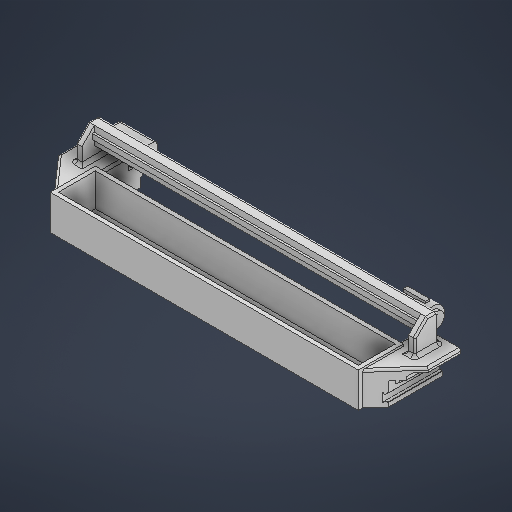
# Autodesk Inventor part: SACMI PH1500 HOPPER FEEDER
Saved by Autodesk Inventor 2025 (Build 290162000, 162)
## iProperties
Created: 2024-05-04
Part Number: SACMI PH1500 HOPPER FEEDER
Material: Generic
Document SubType Name: Modeling
Designer: zulet
Density: 1 g/cm^3
Appearance: Default
Author: zulet
Autodesk Inventor part; units mm, degrees
ref_plane "YZ Plane" through (0, 0, 0) normal (1, 0, 0) x (0, 1, 0)
ref_plane "XZ Plane" through (0, 0, 0) normal (0, 1, 0) x (-1, 0, 0)
ref_plane "XY Plane" through (0, 0, 0) normal (0, 0, 1) x (1, 0, 0)
sketch "Sketch1" plane through (0, 0, 0) normal (0, 1, 0) x (-1, 0, 0)
  line L0 (750, -110) -> (-750, -110)
  line L1 (-750, -110) -> (-750, 110)
  line L2 (-750, 110) -> (750, 110)
  line L3 (750, 110) -> (750, -110)
  line L4 (750, -110) -> (-750, 110) construction
  line L5 (-750, -110) -> (750, 110) construction
  line L6 (-730, -90) -> (730, -90)
  line L7 (730, -90) -> (730, 90)
  line L8 (730, 90) -> (-730, 90)
  line L9 (-730, 90) -> (-730, -90)
  line L10 (-750, 90) -> (-900, -80)
  line L11 (-900, -80) -> (-900, -240)
  line L12 (-900, -240) -> (-720, -240)
  line L13 (-720, -240) -> (-720, -110)
  point P0 (0, 0)
  dimension "d0" = 1500
  dimension "d1" = 220
  dimension "d2" = 20
  dimension "d7" = 150
  dimension "d8" = 20
  dimension "d9" = 30
  dimension "d10" = 130
  dimension "d11" = 30
  constraints: 28 end point, 4 parallel, 4 perpendicular, 2 midpoint, 2 point on line, 1 horizontal, 1 vertical, 3 other
  measures "d0" distance of L1.end L2.end
  measures "d1" distance of L0.end L1.end
  measures "d2" distance between parallel lines of L0 L6
  measures "d7" distance between parallel lines of L11 L1
  measures "d8" distance from line of L2 L10.start
  measures "d9" distance from line of L10.end L0
  measures "d10" distance between parallel lines of L0 L12
  measures "d11" distance between parallel lines of L1 L13
extrude "Extrusion1" add sketch "Sketch1" along normal blind 10 contours L9 L8 L7 L6
extrude "Extrusion2" add sketch "Sketch1" along normal blind 170 contours L0 L1 L2 L3
extrude "Extrusion3" add sketch "Sketch1" along normal blind 160 contours L13 L12 L11 L10 L1 L0
sketch "Sketch2" plane through (900, 0, -240) normal (0, 0, -1) x (-1, 0, 0)
  line L0 (150, 0) -> (0, 0) projected
  line L1 (90, 110) -> (50, 110)
  line L2 (50, 125) -> (35, 140)
  line L3 (35, 140) -> (0, 140)
  line L4 (0, 160) -> (180, 160) projected
  line L5 (0, 0) -> (180, 0) projected
  line L6 (180, 0) -> (180, 160) projected
  line L7 (0, 160) -> (180, 160) projected
  line L8 (0, 0) -> (0, 160) projected
  line L9 (90, 110) -> (90, 0)
  line L10 (65, 110) -> (75, 110)
  line L11 (75, 110) -> (75, 100)
  line L12 (75, 100) -> (65, 100)
  line L13 (65, 100) -> (65, 110)
  line L14 (90, 20) -> (105, 20)
  line L15 (105, 20) -> (105, 60)
  line L16 (105, 60) -> (90, 60)
  line L17 (90, 60) -> (90, 20)
  circle A0 centre (97.5, 60) radius 5
  circle A1 centre (97.5, 20) radius 5
  line L18 (50, 125) -> (50, 110)
  point P0 (900, 0)
  point P1 (70, 110)
  point P2 (90, 20)
  point P3 (92.5, 20)
  point P4 (102.5, 20)
  point P5 (102.5, 60)
  point P6 (92.5, 60)
  point P7 (90, 75.9726)
  point P8 (75, 110)
  point P9 (65, 110)
  point P10 (75, 110)
  dimension "d14" = 20
  dimension "d15" = 35
  dimension "d16" = 15
  dimension "d17" = 15
  dimension "d18" = 40
  dimension "d19" = 10
  dimension "d20" = 10
  dimension "d21" = 15
  dimension "d22" = 40
  dimension "d23" = 10
  dimension "d24" = 10
  dimension "d28" = 15
  dimension "d29" = 50
  constraints: 26 end point, 5 midpoint, 5 parallel, 2 centre point, 2 horizontal, 2 perpendicular, 2 point on line, 1 vertical
  measures "d14" distance between parallel lines of L4 L3
  measures "d15" distance of L2.end L3.end
  measures "d16" horizontal distance of L2.start L2.end
  measures "d17" horizontal distance of L2.start L2.end
  measures "d18" distance of L1.start L1.end
  measures "d19" distance of L11.end L12.end
  measures "d20" distance of L10.end L11.end
  measures "d21" distance of L15.end L16.end
  measures "d22" distance of L14.end L15.end
  measures "d23" diameter of A0
  measures "d24" diameter of A1
  measures "d28" distance of L2.start L1.end
  measures "d29" distance between parallel lines of L1 L16
extrude "Extrusion4" cut sketch "Sketch2" against normal through all contours L0 L8 L3 L2 L18 L1 L13 L12 L11 L9 | L9 L16 A0 L15 L14 A1
fillet "Fillet1" radius 10 3 edges at (825, 160, 5) (900, 160, -160) (720, 160, -175)
mirror "Mirror1" about plane through (0, 0, 0) normal (1, 0, 0) of "Extrusion3", "Extrusion4", "Fillet1"
sketch "Sketch3" plane through (0, 160, 0) normal (0, 1, 0) x (1, 0, 0)
  line L0 (795, 205) -> (825, 205)
  line L1 (825, 205) -> (825, 90)
  line L2 (825, 90) -> (795, 90)
  line L3 (795, 90) -> (795, 205)
  line L4 (890, 240) -> (730, 240) construction
  line L5 (810, 240) -> (810, -10) construction
  line L6 (807.5, 240) -> (807.5, -24.8333) construction
  line L7 (810, 240) -> (1060, 240) construction
  point P0 (0, 0)
  point P1 (810, 205)
  dimension "d30" = 30
  dimension "d31" = 115
  dimension "d32" = 250
  dimension "d33" = 90
  dimension "d34" = 35
  constraints: 12 end point, 3 parallel, 2 horizontal, 2 midpoint, 2 perpendicular, 1 point on line
  measures "d30" distance of L1.end L2.end
  measures "d31" distance of L0.end L1.end
  measures "d32" distance of L5.start L5.end
  measures "d33" angle of L5 L7
  measures "d34" distance between parallel lines of L4 L0
extrude "Extrusion5" add sketch "Sketch3" along normal blind 140
chamfer "Chamfer1" distance 60 angle 45 1 edges at (810, 300, -90)
fillet "Fillet2" radius 8 4 edges at (825, 300, -177.5) (825, 270, -120) (825, 200, -90) (825, 230, -205)
fillet "Fillet3" radius 15 6 edges at (822.6569, 160, -92.3431) (806, 160, -90) (822.6569, 160, -202.6569) (806, 160, -205) (825, 160, -147.5) (795, 160, -147.5)
mirror "Mirror2" about plane through (0, 0, 0) normal (1, 0, 0) of "Extrusion5", "Chamfer1", "Fillet2", "Fillet3"
sketch "Sketch4" plane through (-795, 175, -205) normal (1, 0, 0) x (0, 0, -1)
  line L0 (0, 0) -> (-115, 0) projected
  line L1 (0, 0) -> (0, 125) projected
  line L2 (0, 125) -> (-55, 125) projected
  line L3 (-55, 125) -> (-115, 65) projected
  line L4 (-115, 0) -> (-115, 65) projected
  line L5 (0, 125) -> (0, 0) projected
  line L6 (-55, 125) -> (0, 125)
  line L7 (0, 125) -> (0, 40)
  line L8 (0, 40) -> (-55, 40)
  line L9 (-55, 40) -> (-55, 125)
  line L10 (-55, 95) -> (-65, 95)
  line L11 (-65, 95) -> (-65, 70)
  line L12 (-65, 70) -> (-55, 70)
  line L13 (-55, 70) -> (-55, 95)
  point P0 (-205, -175)
  point P1 (-55, 82.5)
  point P2 (-55, 70)
  point P3 (-55, 95)
  dimension "d42" = 85
  dimension "d45" = 10
  dimension "d46" = 25
  constraints: 16 end point, 4 parallel, 2 horizontal, 2 midpoint, 2 perpendicular, 1 point on line
  measures "d42" distance of L8.end L2.end
  measures "d45" distance of L12.end L11.end
  measures "d46" distance of L11.end L10.end
extrude "Extrusion6" add sketch "Sketch4" along normal up to surface (1590 mm away) contours L8 L9 L2 L1 | L12 L11 L10 L9
chamfer "Chamfer2" distance 30 angle 45 1 edges at (0, 215, -205)
fillet "Fillet4" radius 15 3 edges at (-822.6569, 297.6569, -202.6569) (822.6569, 297.6569, -202.6569) (0, 300, -205)
sketch "Sketch5" plane through (-720, 0, -240) normal (0, 0, -1) x (-1, 0, 0)
  line L0 (-1440, 150) -> (-1440, 0) projected
  line L1 (-1440, 0) -> (-1470, 0)
  line L2 (-1470, 0) -> (-1470, 100)
  line L3 (-1470, 100) -> (-1440, 100)
  line L4 (-1440, 100) -> (-1440, 0)
  line L5 (90, 0) -> (0, 0) projected
  line L6 (0, 0) -> (30, 0)
  line L7 (30, 0) -> (30, 100)
  line L8 (30, 100) -> (0, 100)
  line L9 (0, 100) -> (0, 0)
  point P0 (-720, 0)
  dimension "d51" = 30
  dimension "d52" = 100
  dimension "d53" = 30
  dimension "d54" = 100
  constraints: 16 end point, 4 parallel, 2 horizontal, 2 perpendicular
  measures "d51" distance of L2.end L3.end
  measures "d52" distance of L1.end L2.end
  measures "d53" distance of L8.end L7.end
  measures "d54" distance of L7.end L6.end
extrude "Extrusion7" add sketch "Sketch5" along normal blind 60
sketch "Sketch6" plane through (-720, 0, -300) normal (0, 0, -1) x (-1, 0, 0)
  line L0 (180, 160) -> (0, 160)
  line L1 (0, 160) -> (0, 80)
  line L2 (0, 80) -> (180, 80)
  line L3 (180, 80) -> (180, 160)
  line L4 (170, 160) -> (10, 160) projected
  line L5 (180, 140) -> (180, 150) projected
  point P0 (-720, 0)
  dimension "d57" = 180
  dimension "d58" = 80
  constraints: 8 end point, 2 collinear, 2 parallel, 1 horizontal, 1 perpendicular
  measures "d57" distance of L2.end L1.end
  measures "d58" distance of L1.end L0.end
extrude "Extrusion8" add sketch "Sketch6" along normal blind 80
fillet "Fillet5" radius 15 8 edges at (-810, 160, -380) (-900, 160, -340) (-810, 160, -300) (-900, 120, -300) (-900, 120, -380) (-900, 80, -340) (-810, 80, -380) (-825, 80, -300)
chamfer "Chamfer3" distance 40 angle 45 1 edges at (-735, 100, -300)
chamfer "Chamfer4" distance 40 angle 45 1 edges at (-735, 80, -300)
fillet "Fillet6" radius 10 3 edges at (-750, 84.3934, -304.3934) (-750, 80, -327.5) (-750, 117.5, -300)
sketch "Sketch7" plane through (-720, 0, -110) normal (1, 0, 0) x (0, 0, -1)
  line L0 (205, 145) -> (205, 95) projected
  line L1 (255, 95) -> (255, 80) projected
  line L2 (205, 145) -> (255, 95) construction
  line L3 (255, 145) -> (270, 145) projected
  line L4 (205, 95) -> (255, 95) projected
  line L5 (255, 145) -> (205, 95) construction
  circle A0 centre (230, 120) radius 25
  line L6 (255, 145) -> (205, 145) projected
  point P0 (-110, 0)
  constraints: 4 end point, 1 centre point, 1 midpoint, 1 tangent
extrude "Extrusion9" add sketch "Sketch7" along normal blind 1250 contours A0
sketch "Sketch8" plane through (530, 120, -340) normal (1, 0, 0) x (0, 0, -1)
  circle A0 centre (0, 0) radius 25 projected
  circle A1 centre (0, 0) radius 50
  point P0 (-340, -120)
  dimension "d71" = 100
  constraints: 1 centre point, 1 coincident
  measures "d71" diameter of A1
extrude "Extrusion10" add sketch "Sketch8" along normal blind 15 contours A0 | A1
sketch "Sketch9" plane through (545, 120, -340) normal (1, 0, 0) x (0, 0, -1)
  circle A0 centre (0, 0) radius 50 projected
  line L0 (2, 57.5) -> (-2, 57.5)
  line L1 (-2, 57.5) -> (-2, 44.5)
  line L2 (0, 42.5) -> (0, 42.5)
  line L3 (2, 44.5) -> (2, 57.5)
  line L4 (2, 57.5) -> (-2, 42.5) construction
  line L5 (-2, 57.5) -> (2, 42.5) construction
  arc A1 (-2, 44.5) -> (0, 42.5) centre (0, 44.5) ccw
  arc A2 (0, 42.5) -> (2, 44.5) centre (0, 44.5) ccw
  line L6 (-12.2349, 56.2188) -> (-9.9136, 43.4278)
  arc A3 (-9.9136, 43.4278) -> (-7.5887, 41.817) centre (-7.9458, 43.7849) ccw
  arc A4 (-7.5887, 41.817) -> (-5.9779, 44.142) centre (-7.9458, 43.7849) ccw
  line L7 (-5.9779, 44.142) -> (-8.2992, 56.9331)
  line L8 (-8.2992, 56.9331) -> (-12.2349, 56.2188)
  line L9 (-22.0765, 53.1308) -> (-17.5086, 40.9597)
  arc A5 (-17.5086, 40.9597) -> (-14.9334, 39.79) centre (-15.6362, 41.6625) ccw
  arc A6 (-14.9334, 39.79) -> (-13.7637, 42.3652) centre (-15.6362, 41.6625) ccw
  line L10 (-13.7637, 42.3652) -> (-18.3316, 54.5363)
  line L11 (-18.3316, 54.5363) -> (-22.0765, 53.1308)
  line L12 (-31.2086, 48.335) -> (-24.5409, 37.1752)
  arc A7 (-24.5409, 37.1752) -> (-21.7982, 36.4841) centre (-22.824, 38.201) ccw
  arc A8 (-21.7982, 36.4841) -> (-21.1071, 39.2268) centre (-22.824, 38.201) ccw
  line L13 (-21.1071, 39.2268) -> (-27.7748, 50.3866)
  line L14 (-27.7748, 50.3866) -> (-31.2086, 48.335)
  line L15 (-39.3376, 41.9857) -> (-30.7844, 32.1958)
  arc A9 (-30.7844, 32.1958) -> (-27.9624, 32.0055) centre (-29.2783, 33.5117) ccw
  arc A10 (-27.9624, 32.0055) -> (-27.7721, 34.8276) centre (-29.2783, 33.5117) ccw
  line L16 (-27.7721, 34.8276) -> (-36.3253, 44.6175)
  line L17 (-36.3253, 44.6175) -> (-39.3376, 41.9857)
  line L18 (-46.2023, 34.287) -> (-36.0385, 26.1816)
  arc A11 (-36.0385, 26.1816) -> (-33.2278, 26.4983) centre (-34.7915, 27.7453) ccw
  arc A12 (-33.2278, 26.4983) -> (-33.5445, 29.309) centre (-34.7915, 27.7453) ccw
  line L19 (-33.5445, 29.309) -> (-43.7083, 37.4143)
  line L20 (-43.7083, 37.4143) -> (-46.2023, 34.287)
  line L21 (-51.582, 25.4863) -> (-40.1342, 19.326)
  arc A13 (-40.1342, 19.326) -> (-37.4253, 20.1394) centre (-39.1865, 21.0872) ccw
  arc A14 (-37.4253, 20.1394) -> (-38.2388, 22.8483) centre (-39.1865, 21.0872) ccw
  line L22 (-38.2388, 22.8483) -> (-49.6865, 29.0086)
  line L23 (-49.6865, 29.0086) -> (-51.582, 25.4863)
  line L24 (-55.3038, 15.8664) -> (-42.94, 11.8491)
  arc A15 (-42.94, 11.8491) -> (-40.4199, 13.1332) centre (-42.322, 13.7513) ccw
  arc A16 (-40.4199, 13.1332) -> (-41.704, 15.6534) centre (-42.322, 13.7513) ccw
  line L25 (-41.704, 15.6534) -> (-54.0677, 19.6706)
  line L26 (-54.0677, 19.6706) -> (-55.3038, 15.8664)
  line L27 (-57.2481, 5.7365) -> (-44.3657, 3.9915)
  arc A17 (-44.3657, 3.9915) -> (-42.1154, 5.7049) centre (-44.0973, 5.9734) ccw
  arc A18 (-42.1154, 5.7049) -> (-43.8288, 7.9553) centre (-44.0973, 5.9734) ccw
  line L28 (-43.8288, 7.9553) -> (-56.7111, 9.7003)
  line L29 (-56.7111, 9.7003) -> (-57.2481, 5.7365)
  line L30 (-57.3524, -4.5777) -> (-44.3655, -3.9945)
  arc A19 (-44.3655, -3.9945) -> (-42.4572, -1.9068) centre (-44.4552, -1.9965) ccw
  arc A20 (-42.4572, -1.9068) -> (-44.5449, 0.0015) centre (-44.4552, -1.9965) ccw
  line L31 (-44.5449, 0.0015) -> (-57.5318, -0.5817)
  line L32 (-57.5318, -0.5817) -> (-57.3524, -4.5777)
  line L33 (-55.6133, -14.7448) -> (-42.9393, -11.852)
  arc A21 (-42.9393, -11.852) -> (-41.4344, -9.4571) centre (-43.3843, -9.9022) ccw
  arc A22 (-41.4344, -9.4571) -> (-43.8293, -7.9523) centre (-43.3843, -9.9022) ccw
  line L34 (-43.8293, -7.9523) -> (-56.5034, -10.8451)
  line L35 (-56.5034, -10.8451) -> (-55.6133, -14.7448)
  line L36 (-52.0868, -24.438) -> (-40.1329, -19.3287)
  arc A23 (-40.1329, -19.3287) -> (-39.0799, -16.7036) centre (-40.919, -17.4896) ccw
  arc A24 (-39.0799, -16.7036) -> (-41.705, -15.6506) centre (-40.919, -17.4896) ccw
  line L37 (-41.705, -15.6506) -> (-53.6589, -20.7599)
  line L38 (-53.6589, -20.7599) -> (-52.0868, -24.438)
  line L39 (-46.8862, -33.3457) -> (-36.0367, -26.1841)
  arc A25 (-36.0367, -26.1841) -> (-35.4694, -23.4131) centre (-37.1385, -24.5149) ccw
  arc A26 (-35.4694, -23.4131) -> (-38.2403, -22.8458) centre (-37.1385, -24.5149) ccw
  line L40 (-38.2403, -22.8458) -> (-49.0898, -30.0074)
  line L41 (-49.0898, -30.0074) -> (-46.8862, -33.3457)
  line L42 (-40.1786, -41.1817) -> (-30.7822, -32.1979)
  arc A27 (-30.7822, -32.1979) -> (-30.7188, -29.3702) centre (-32.1644, -30.7523) ccw
  arc A28 (-30.7188, -29.3702) -> (-33.5465, -29.3067) centre (-32.1644, -30.7523) ccw
  line L43 (-33.5465, -29.3067) -> (-42.9428, -38.2905)
  line L44 (-42.9428, -38.2905) -> (-40.1786, -41.1817)
  line L45 (-32.1796, -47.694) -> (-24.5384, -37.1768)
  arc A29 (-24.5384, -37.1768) -> (-24.9809, -34.3832) centre (-26.1564, -36.0013) ccw
  arc A30 (-24.9809, -34.3832) -> (-27.7745, -34.8257) centre (-26.1564, -36.0013) ccw
  line L46 (-27.7745, -34.8257) -> (-35.4157, -45.3429)
  line L47 (-35.4157, -45.3429) -> (-32.1796, -47.694)
  line L48 (-23.1464, -52.6735) -> (-17.5059, -40.9609)
  arc A31 (-17.5059, -40.9609) -> (-18.4401, -38.2912) centre (-19.3078, -40.0931) ccw
  arc A32 (-18.4401, -38.2912) -> (-21.1098, -39.2253) centre (-19.3078, -40.0931) ccw
  line L49 (-21.1098, -39.2253) -> (-26.7503, -50.9379)
  line L50 (-26.7503, -50.9379) -> (-23.1464, -52.6735)
  line L51 (-13.3692, -55.9599) -> (-9.9107, -43.4284)
  arc A33 (-9.9107, -43.4284) -> (-11.3066, -40.9684) centre (-11.8386, -42.8963) ccw
  arc A34 (-11.3066, -40.9684) -> (-13.7666, -42.3643) centre (-11.8386, -42.8963) ccw
  line L52 (-13.7666, -42.3643) -> (-17.225, -54.8958)
  line L53 (-17.225, -54.8958) -> (-13.3692, -55.9599)
  line L54 (-3.1623, -57.4478) -> (-1.997, -44.5001)
  arc A35 (-1.997, -44.5001) -> (-3.8097, -42.3289) centre (-3.9889, -44.3209) ccw
  arc A36 (-3.8097, -42.3289) -> (-5.9809, -44.1416) centre (-3.9889, -44.3209) ccw
  line L55 (-5.9809, -44.1416) -> (-7.1462, -57.0892)
  line L56 (-7.1462, -57.0892) -> (-3.1623, -57.4478)
  line L57 (7.1462, -57.0892) -> (5.9809, -44.1416)
  arc A37 (5.9809, -44.1416) -> (3.8097, -42.3289) centre (3.9889, -44.3209) ccw
  arc A38 (3.8097, -42.3289) -> (1.997, -44.5001) centre (3.9889, -44.3209) ccw
  line L58 (1.997, -44.5001) -> (3.1623, -57.4478)
  line L59 (3.1623, -57.4478) -> (7.1462, -57.0892)
  line L60 (17.225, -54.8958) -> (13.7666, -42.3643)
  arc A39 (13.7666, -42.3643) -> (11.3066, -40.9684) centre (11.8386, -42.8963) ccw
  arc A40 (11.3066, -40.9684) -> (9.9107, -43.4284) centre (11.8386, -42.8963) ccw
  line L61 (9.9107, -43.4284) -> (13.3692, -55.9599)
  line L62 (13.3692, -55.9599) -> (17.225, -54.8958)
  line L63 (26.7503, -50.9379) -> (21.1098, -39.2253)
  arc A41 (21.1098, -39.2253) -> (18.4401, -38.2912) centre (19.3078, -40.0931) ccw
  arc A42 (18.4401, -38.2912) -> (17.5059, -40.9609) centre (19.3078, -40.0931) ccw
  line L64 (17.5059, -40.9609) -> (23.1464, -52.6735)
  line L65 (23.1464, -52.6735) -> (26.7503, -50.9379)
  line L66 (35.4157, -45.3429) -> (27.7745, -34.8257)
  arc A43 (27.7745, -34.8257) -> (24.9809, -34.3832) centre (26.1564, -36.0013) ccw
  arc A44 (24.9809, -34.3832) -> (24.5384, -37.1768) centre (26.1564, -36.0013) ccw
  line L67 (24.5384, -37.1768) -> (32.1796, -47.694)
  line L68 (32.1796, -47.694) -> (35.4157, -45.3429)
  line L69 (42.9428, -38.2905) -> (33.5465, -29.3067)
  arc A45 (33.5465, -29.3067) -> (30.7188, -29.3702) centre (32.1644, -30.7523) ccw
  arc A46 (30.7188, -29.3702) -> (30.7822, -32.1979) centre (32.1644, -30.7523) ccw
  line L70 (30.7822, -32.1979) -> (40.1786, -41.1817)
  line L71 (40.1786, -41.1817) -> (42.9428, -38.2905)
  line L72 (49.0898, -30.0074) -> (38.2403, -22.8458)
  arc A47 (38.2403, -22.8458) -> (35.4694, -23.4131) centre (37.1385, -24.5149) ccw
  arc A48 (35.4694, -23.4131) -> (36.0367, -26.1841) centre (37.1385, -24.5149) ccw
  line L73 (36.0367, -26.1841) -> (46.8862, -33.3457)
  line L74 (46.8862, -33.3457) -> (49.0898, -30.0074)
  line L75 (53.6589, -20.7599) -> (41.705, -15.6506)
  arc A49 (41.705, -15.6506) -> (39.0799, -16.7036) centre (40.919, -17.4896) ccw
  arc A50 (39.0799, -16.7036) -> (40.1329, -19.3287) centre (40.919, -17.4896) ccw
  line L76 (40.1329, -19.3287) -> (52.0868, -24.438)
  line L77 (52.0868, -24.438) -> (53.6589, -20.7599)
  line L78 (56.5034, -10.8451) -> (43.8293, -7.9523)
  arc A51 (43.8293, -7.9523) -> (41.4344, -9.4571) centre (43.3843, -9.9022) ccw
  arc A52 (41.4344, -9.4571) -> (42.9393, -11.852) centre (43.3843, -9.9022) ccw
  line L79 (42.9393, -11.852) -> (55.6133, -14.7448)
  line L80 (55.6133, -14.7448) -> (56.5034, -10.8451)
  line L81 (57.5318, -0.5817) -> (44.5449, 0.0015)
  arc A53 (44.5449, 0.0015) -> (42.4572, -1.9068) centre (44.4552, -1.9965) ccw
  arc A54 (42.4572, -1.9068) -> (44.3655, -3.9945) centre (44.4552, -1.9965) ccw
  line L82 (44.3655, -3.9945) -> (57.3524, -4.5777)
  line L83 (57.3524, -4.5777) -> (57.5318, -0.5817)
  line L84 (56.7111, 9.7003) -> (43.8288, 7.9553)
  arc A55 (43.8288, 7.9553) -> (42.1154, 5.7049) centre (44.0973, 5.9734) ccw
  arc A56 (42.1154, 5.7049) -> (44.3657, 3.9915) centre (44.0973, 5.9734) ccw
  line L85 (44.3657, 3.9915) -> (57.2481, 5.7365)
  line L86 (57.2481, 5.7365) -> (56.7111, 9.7003)
  line L87 (54.0677, 19.6706) -> (41.704, 15.6534)
  arc A57 (41.704, 15.6534) -> (40.4199, 13.1332) centre (42.322, 13.7513) ccw
  arc A58 (40.4199, 13.1332) -> (42.94, 11.8491) centre (42.322, 13.7513) ccw
  line L88 (42.94, 11.8491) -> (55.3038, 15.8664)
  line L89 (55.3038, 15.8664) -> (54.0677, 19.6706)
  line L90 (49.6865, 29.0086) -> (38.2388, 22.8483)
  arc A59 (38.2388, 22.8483) -> (37.4253, 20.1394) centre (39.1865, 21.0872) ccw
  arc A60 (37.4253, 20.1394) -> (40.1342, 19.326) centre (39.1865, 21.0872) ccw
  line L91 (40.1342, 19.326) -> (51.582, 25.4863)
  line L92 (51.582, 25.4863) -> (49.6865, 29.0086)
  line L93 (43.7083, 37.4143) -> (33.5445, 29.309)
  arc A61 (33.5445, 29.309) -> (33.2278, 26.4983) centre (34.7915, 27.7453) ccw
  arc A62 (33.2278, 26.4983) -> (36.0385, 26.1816) centre (34.7915, 27.7453) ccw
  line L94 (36.0385, 26.1816) -> (46.2023, 34.287)
  line L95 (46.2023, 34.287) -> (43.7083, 37.4143)
  line L96 (36.3253, 44.6175) -> (27.7721, 34.8276)
  arc A63 (27.7721, 34.8276) -> (27.9624, 32.0055) centre (29.2783, 33.5117) ccw
  arc A64 (27.9624, 32.0055) -> (30.7844, 32.1958) centre (29.2783, 33.5117) ccw
  line L97 (30.7844, 32.1958) -> (39.3376, 41.9857)
  line L98 (39.3376, 41.9857) -> (36.3253, 44.6175)
  line L99 (27.7748, 50.3866) -> (21.1071, 39.2268)
  arc A65 (21.1071, 39.2268) -> (21.7982, 36.4841) centre (22.824, 38.201) ccw
  arc A66 (21.7982, 36.4841) -> (24.5409, 37.1752) centre (22.824, 38.201) ccw
  line L100 (24.5409, 37.1752) -> (31.2086, 48.335)
  line L101 (31.2086, 48.335) -> (27.7748, 50.3866)
  line L102 (18.3316, 54.5363) -> (13.7637, 42.3652)
  arc A67 (13.7637, 42.3652) -> (14.9334, 39.79) centre (15.6362, 41.6625) ccw
  arc A68 (14.9334, 39.79) -> (17.5086, 40.9597) centre (15.6362, 41.6625) ccw
  line L103 (17.5086, 40.9597) -> (22.0765, 53.1308)
  line L104 (22.0765, 53.1308) -> (18.3316, 54.5363)
  line L105 (8.2992, 56.9331) -> (5.9779, 44.142)
  arc A69 (5.9779, 44.142) -> (7.5887, 41.817) centre (7.9458, 43.7849) ccw
  arc A70 (7.5887, 41.817) -> (9.9136, 43.4278) centre (7.9458, 43.7849) ccw
  line L106 (9.9136, 43.4278) -> (12.2349, 56.2188)
  line L107 (12.2349, 56.2188) -> (8.2992, 56.9331)
  point P0 (-340, -120)
  point P1 (0, 50)
  point P2 (-9.5565, 41.4599)
  point P3 (-5.6208, 42.1741)
  point P4 (-16.8059, 39.0872)
  point P5 (-13.061, 40.4927)
  point P6 (-23.5151, 35.4583)
  point P7 (-20.0813, 37.5099)
  point P8 (-29.4685, 30.6897)
  point P9 (-26.4563, 33.3214)
  point P10 (-34.4748, 24.9347)
  point P11 (-31.9809, 28.062)
  point P12 (-38.373, 18.3782)
  point P13 (-36.4776, 21.9006)
  point P14 (-41.0379, 11.2311)
  point P15 (-39.8019, 15.0353)
  point P16 (-42.3838, 3.723)
  point P17 (-41.8469, 7.6868)
  point P18 (-42.3675, -3.9047)
  point P19 (-42.5469, 0.0912)
  point P20 (-40.9894, -11.407)
  point P21 (-41.8795, -7.5073)
  point P22 (-38.2939, -18.5426)
  point P23 (-39.866, -14.8645)
  point P24 (-34.3676, -25.0823)
  point P25 (-36.5712, -21.744)
  point P26 (-29.3367, -30.8158)
  point P27 (-32.1009, -27.9246)
  point P28 (-23.3628, -35.5588)
  point P29 (-26.5989, -33.2077)
  point P30 (-16.6381, -39.1589)
  point P31 (-20.242, -37.4234)
  point P32 (-9.3786, -41.5005)
  point P33 (-13.2345, -40.4363)
  point P34 (-1.8177, -42.5082)
  point P35 (-5.8016, -42.1496)
  point P36 (5.8016, -42.1496)
  point P37 (1.8177, -42.5082)
  point P38 (13.2345, -40.4363)
  point P39 (9.3786, -41.5005)
  point P40 (20.242, -37.4234)
  point P41 (16.6381, -39.1589)
  point P42 (26.5989, -33.2077)
  point P43 (23.3628, -35.5588)
  point P44 (32.1009, -27.9246)
  point P45 (29.3367, -30.8158)
  point P46 (36.5712, -21.744)
  point P47 (34.3676, -25.0823)
  point P48 (39.866, -14.8645)
  point P49 (38.2939, -18.5426)
  point P50 (41.8795, -7.5073)
  point P51 (40.9894, -11.407)
  point P52 (42.5469, 0.0912)
  point P53 (42.3675, -3.9047)
  point P54 (41.8469, 7.6868)
  point P55 (42.3838, 3.723)
  point P56 (39.8019, 15.0353)
  point P57 (41.0379, 11.2311)
  point P58 (36.4776, 21.9006)
  point P59 (38.373, 18.3782)
  point P60 (31.9809, 28.062)
  point P61 (34.4748, 24.9347)
  point P62 (26.4563, 33.3214)
  point P63 (29.4685, 30.6897)
  point P64 (20.0813, 37.5099)
  point P65 (23.5151, 35.4583)
  point P66 (13.061, 40.4927)
  point P67 (16.8059, 39.0872)
  point P68 (5.6208, 42.1741)
  point P69 (9.5565, 41.4599)
  point P70 (0, 42.5)
  point P71 (-2, 49.96)
  point P72 (-6.9528, 49.5142)
  point P73 (-7.5887, 41.817)
  point P74 (-10.8886, 48.8)
  point P75 (-15.6822, 47.477)
  point P76 (-14.9334, 39.79)
  point P77 (-19.4272, 46.0715)
  point P78 (-23.9075, 43.9139)
  point P79 (-21.7982, 36.4841)
  point P80 (-27.3413, 41.8623)
  point P81 (-31.3645, 38.9393)
  point P82 (-27.9624, 32.0055)
  point P83 (-34.3768, 36.3076)
  point P84 (-37.8133, 32.7132)
  point P85 (-33.2278, 26.4983)
  point P86 (-40.3073, 29.5859)
  point P87 (-43.0468, 25.4357)
  point P88 (-37.4253, 20.1394)
  point P89 (-44.9423, 21.9133)
  point P90 (-46.8967, 17.3406)
  point P91 (-40.4199, 13.1332)
  point P92 (-48.1328, 13.5364)
  point P93 (-49.2394, 8.6882)
  point P94 (-42.1154, 5.7049)
  point P95 (-49.7763, 4.7244)
  point P96 (-49.9994, -0.2435)
  point P97 (-42.4572, -1.9068)
  point P98 (-49.8199, -4.2394)
  point P99 (-49.1524, -9.1673)
  point P100 (-48.2623, -13.067)
  point P101 (-46.7256, -17.7965)
  point P102 (-39.0799, -16.7036)
  point P103 (-45.1535, -21.4746)
  point P104 (-42.7971, -25.8537)
  point P105 (-35.4694, -23.4131)
  point P106 (-40.5935, -29.192)
  point P107 (-37.4929, -33.0799)
  point P108 (-30.7188, -29.3702)
  point P109 (-34.7287, -35.9711)
  point P110 (-30.9838, -39.2429)
  point P111 (-24.9809, -34.3832)
  point P112 (-27.7477, -41.594)
  point P113 (-23.4788, -44.1446)
  point P114 (-18.4401, -38.2912)
  point P115 (-19.8749, -45.8802)
  point P116 (-15.2191, -47.6275)
  point P117 (-11.3066, -40.9684)
  point P118 (-11.3633, -48.6916)
  point P119 (-6.4703, -49.5796)
  point P120 (-3.8097, -42.3289)
  point P121 (-2.4864, -49.9381)
  point P122 (2.4864, -49.9381)
  point P123 (3.8097, -42.3289)
  point P124 (6.4703, -49.5796)
  point P125 (11.3633, -48.6916)
  point P126 (11.3066, -40.9684)
  point P127 (15.2191, -47.6275)
  point P128 (19.8749, -45.8802)
  point P129 (18.4401, -38.2912)
  point P130 (23.4788, -44.1446)
  point P131 (27.7477, -41.594)
  point P132 (24.9809, -34.3832)
  point P133 (30.9838, -39.2429)
  point P134 (34.7287, -35.9711)
  point P135 (30.7188, -29.3702)
  point P136 (37.4929, -33.0799)
  point P137 (40.5935, -29.192)
  point P138 (35.4694, -23.4131)
  point P139 (42.7971, -25.8537)
  point P140 (45.1535, -21.4746)
  point P141 (39.0799, -16.7036)
  point P142 (46.7256, -17.7965)
  point P143 (48.2623, -13.067)
  point P144 (41.4344, -9.4571)
  point P145 (49.1524, -9.1673)
  point P146 (49.8199, -4.2394)
  point P147 (42.4572, -1.9068)
  point P148 (49.9994, -0.2435)
  point P149 (49.7763, 4.7244)
  point P150 (42.1154, 5.7049)
  point P151 (49.2394, 8.6882)
  point P152 (48.1328, 13.5364)
  point P153 (40.4199, 13.1332)
  point P154 (46.8967, 17.3406)
  point P155 (44.9423, 21.9133)
  point P156 (37.4253, 20.1394)
  point P157 (43.0468, 25.4357)
  point P158 (40.3073, 29.5859)
  point P159 (33.2278, 26.4983)
  point P160 (37.8133, 32.7132)
  point P161 (34.3768, 36.3076)
  point P162 (27.9624, 32.0055)
  point P163 (31.3645, 38.9393)
  point P164 (27.3413, 41.8623)
  point P165 (21.7982, 36.4841)
  point P166 (23.9075, 43.9139)
  point P167 (19.4272, 46.0715)
  point P168 (14.9334, 39.79)
  point P169 (15.6822, 47.477)
  point P170 (10.8886, 48.8)
  point P171 (7.5887, 41.817)
  point P172 (6.9528, 49.5142)
  point P173 (2, 49.96)
  dimension "d74" = 4
  dimension "d75" = 15
  dimension "d76" = 2
  dimension "d79" = 360
  constraints: 216 end point, 140 point on circle, 72 point on line, 70 centre point, 4 tangent, 2 midpoint, 2 parallel, 1 concentric, 1 horizontal, 1 perpendicular, 528 other
  measures "d74" distance of L5.end L4.end
  measures "d75" distance of L4.end L0.end
  measures "d76" radius of A1
extrude "Extrusion11" add sketch "Sketch9" along normal blind 50 contours A0 L81 A53 A54 L82 L78 A51 A52 L79 L75 A49 A50 L76 L72 A47 A48 L73 L69 A45 A46 L70 L66 A43 A44 L67 L63 A41 A42 L64 L60 A39 A40 L61 L57 A37 A38 L58 L54 A35 A36 L55 L51 A33 A34 L52 L48 A31 A32 L49 L45 A29 A30 L46 L42 A27 A28 L43 L39 A25 A26 L40 L36 A23 A24 L37 L33 A21 A22 L34 L30 A19 A20 L31 L27 A17 A18 L28 L24 A15 A16 L25 L21 A13 A14 L22 L18 A11 A12 L19 L15 A9 A10 L16 L12 A7 A8 L13 L9 A5 A6 L10 L6 A3 A4 L7 L1 A1 A2 L3 L105 A69 A70 L106 L102 A67 A68 L103 L99 A65 A66 L100 L96 A63 A64 L97 L93 A61 A62 L94 L90 A59 A60 L91 L87 A57 A58 L88 L84 A55 A56 L85
sketch "Sketch10" plane through (595, 120, -340) normal (1, 0, 0) x (0, 0, -1)
  circle A0 centre (0, 0) radius 50 projected
  circle A1 centre (0, 0) radius 54
  point P0 (-340, -120)
  dimension "d83" = 4
  constraints: 1 centre point
  measures "d83" radial gap between concentric circles of A0 A1
extrude "Extrusion12" add sketch "Sketch10" along normal blind 70.75 contours A0 | A1
sketch "Sketch11" plane through (665.75, 120, -340) normal (1, 0, 0) x (0, 0, -1)
  circle A0 centre (0, 0) radius 25 projected
  circle A1 centre (0, 0) radius 37.5
  point P0 (-340, -120)
  dimension "d86" = 75
  constraints: 1 centre point, 1 coincident
  measures "d86" diameter of A1
extrude "Extrusion13" add sketch "Sketch11" along normal blind 15.5 contours A0 | A1
sketch "Sketch12" plane through (530, 120, -340) normal (-1, 0, 0) x (0, 0, 1)
  arc A0 (-10.8886, 48.8) -> (-15.6822, 47.477) centre (0, 0) ccw projected
  line L0 (-10.8886, 48.8) -> (11.1114, 48.8)
  line L1 (11.1114, 48.8) -> (11.1114, 63.8)
  line L2 (11.1114, 63.8) -> (-10.8886, 63.8)
  line L3 (-10.8886, 63.8) -> (-10.8886, 48.8)
  point P0 (340, -120)
  dimension "d89" = 22
  dimension "d90" = 15
  constraints: 8 end point, 2 parallel, 1 horizontal, 1 perpendicular
  measures "d89" distance of L2.end L1.end
  measures "d90" distance of L1.end L0.end
extrude "Extrusion14" add sketch "Sketch12" against normal blind 107
body "Solid1"
